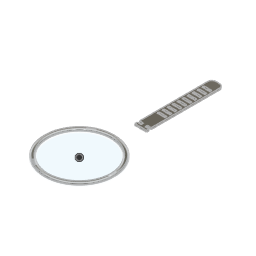
tpuStrapv4 (Autodesk Fusion 360 design; units mm, degrees)
Autodesk Fusion 360 part; units mm, degrees
sketch "Sketch1" plane through (0, 0, 0) normal (0, 0, 1) x (1, 0, 0)
  circle A0 centre (0, 0) radius 40
  circle A1 centre (0, 0) radius 45
  dimension "d1" = 80
  dimension "d3" = 5
  constraint coincident A0.centre A1.centre
  measures "d1" diameter of A0
  measures "d3" distance of A0 A1
extrude "Extrude1" add sketch "Sketch1" along normal blind 3 makes body 1
ref_plane "WorkPlane1" through (60, 0, 0) normal (1, 0, 0) x (0, 1, 0)
sketch "Sketch9" plane through (0, 0, 0) normal (0, 0, 1) x (1, 0, 0)
  circle A0 centre (0, 0) radius 45
  line L0 (-18.1458, 39.7599) -> (-25.3567, 35.5828)
  line L1 (-25.3567, 35.5828) -> (-24.3542, 33.8522)
  line L2 (-24.3542, 33.8522) -> (-17.1433, 38.0293)
  line L3 (-17.1433, 38.0293) -> (-18.1458, 39.7599)
  line L4 (-18.1458, 39.7599) -> (-24.3542, 33.8522) construction
  line L5 (-25.3567, 35.5828) -> (-17.1433, 38.0293) construction
  line L6 (43.5, 4.1667) -> (41.5, 4.1667)
  line L7 (41.5, 4.1667) -> (41.5, -4.1667)
  line L8 (41.5, -4.1667) -> (43.5, -4.1667)
  line L9 (43.5, -4.1667) -> (43.5, 4.1667)
  line L10 (43.5, 4.1667) -> (41.5, -4.1667) construction
  line L11 (41.5, 4.1667) -> (43.5, -4.1667) construction
  line L12 (-17.1416, -38.0234) -> (-18.1416, -39.7554)
  line L13 (-18.1416, -39.7554) -> (-25.3584, -35.5888)
  line L14 (-25.3584, -35.5888) -> (-24.3584, -33.8567)
  line L15 (-24.3584, -33.8567) -> (-17.1416, -38.0234)
  line L16 (-17.1416, -38.0234) -> (-25.3584, -35.5888) construction
  line L17 (-18.1416, -39.7554) -> (-24.3584, -33.8567) construction
  line L18 (0, 0) -> (115, 0)
  line L19 (0, 0) -> (-50, -86.6025)
  line L20 (0, 0) -> (99.9995, 0) construction
  line L21 (0, 0) -> (-50, 86.6025)
  line L22 (0, 0) -> (100, 0) construction
  point P0 (-21.25, 36.8061)
  point P1 (42.5, 0)
  point P2 (-21.25, -36.8061)
  dimension "d44" = 8.3333
  dimension "d45" = 2
  dimension "d46" = 2
  dimension "d47" = 8.3333
  dimension "d48" = 2
  dimension "d49" = 8.3333
  dimension "d108" = 42.5
  dimension "d110" = 42.5
  dimension "d112" = 120
  dimension "d114" = 42.5
  dimension "d115" = 120
  constraint perpendicular L0 L1
  constraint parallel L0 L2
  constraint parallel L1 L3
  constraint coincident L4 P0
  constraint coincident L5 P0
  constraint horizontal L6
  constraint perpendicular L6 L7
  constraint parallel L6 L8
  constraint parallel L7 L9
  constraint coincident L10 P1
  constraint coincident L11 P1
  constraint perpendicular L12 L13
  constraint parallel L12 L14
  constraint parallel L13 L15
  constraint coincident L16 P2
  constraint coincident L17 P2
  constraint coincident A0.centre L18.start
  constraint perpendicular L9 L18
  constraint coincident P1 L18
  constraint horizontal L20
  constraint perpendicular L13 L19
  constraint coincident P2 L19
  constraint horizontal L22
  constraint coincident P0 L21
  measures "d44" distance of L1.end L2.end
  measures "d45" distance of L0.end L1.end
  measures "d46" distance of L7.end L8.end
  measures "d47" distance of L6.end L7.end
  measures "d48" distance of L13.end L14.end
  measures "d49" distance of L12.end L13.end
  measures "d108" distance of P1 A0.centre
  measures "d110" distance of P0 A0.centre
  measures "d112" angle of L19 L20
  measures "d114" distance of P2 A0.centre
  measures "d115" angle of L21 L22
extrude "Extrude3" cut sketch "Sketch9" along normal blind 3 contours L12 L13 L15 L19 | L13 L14 L15 L19 bodies 1
extrude "Extrude4" cut sketch "Sketch9" along normal blind 3 contours L6 L7 L9 L18 | L7 L8 L9 L18 bodies 1
extrude "Extrude5" cut sketch "Sketch9" along normal blind 3 contours L0 L1 L2 L21 | L0 L2 L3 L21 bodies 1
sketch "Sketch10" plane through (0, 0, 0) normal (0, 0, 1) x (1, 0, 0)
  line L0 (15.004, 121.2433) -> (0.004, 121.2433)
  line L1 (0.004, 121.2433) -> (0.004, 124.2433)
  line L2 (0.004, 124.2433) -> (15.004, 124.2433)
  line L3 (15.004, 124.2433) -> (15.004, 121.2433)
  line L4 (10.004, 124.2433) -> (5.004, 124.2433)
  line L5 (5.004, 124.2433) -> (5.004, 127.2433)
  line L6 (5.004, 127.2433) -> (10.004, 127.2433)
  line L7 (10.004, 127.2433) -> (10.004, 124.2433)
  line L8 (15.004, 127.2433) -> (0.004, 127.2433)
  line L9 (0.004, 127.2433) -> (0.004, 214.8433)
  line L10 (5.004, 219.8433) -> (10.004, 219.8433)
  line L11 (15.004, 214.8433) -> (15.004, 127.2433)
  arc A0 (15.004, 214.8433) -> (10.004, 219.8433) centre (10.004, 214.8433) ccw
  arc A1 (5.004, 219.8433) -> (0.004, 214.8433) centre (5.004, 214.8433) ccw
  line L12 (2.504, 147.2433) -> (12.504, 147.2433)
  line L13 (12.504, 147.2433) -> (12.504, 149.6433)
  line L14 (12.504, 149.6433) -> (2.504, 149.6433)
  line L15 (2.504, 149.6433) -> (2.504, 147.2433)
  line L16 (2.504, 147.2433) -> (12.504, 149.6433) construction
  line L17 (12.504, 147.2433) -> (2.504, 149.6433) construction
  line L18 (2.504, 153.6433) -> (12.504, 153.6433)
  line L19 (2.504, 156.0433) -> (2.504, 153.6433)
  line L20 (12.504, 156.0433) -> (2.504, 156.0433)
  line L21 (12.504, 153.6433) -> (12.504, 156.0433)
  line L22 (2.504, 160.0433) -> (12.504, 160.0433)
  line L23 (2.504, 162.4433) -> (2.504, 160.0433)
  line L24 (12.504, 162.4433) -> (2.504, 162.4433)
  line L25 (12.504, 160.0433) -> (12.504, 162.4433)
  line L26 (2.504, 166.4433) -> (12.504, 166.4433)
  line L27 (2.504, 168.8433) -> (2.504, 166.4433)
  line L28 (12.504, 168.8433) -> (2.504, 168.8433)
  line L29 (12.504, 166.4433) -> (12.504, 168.8433)
  line L30 (2.504, 172.8433) -> (12.504, 172.8433)
  line L31 (2.504, 175.2433) -> (2.504, 172.8433)
  line L32 (12.504, 175.2433) -> (2.504, 175.2433)
  line L33 (12.504, 172.8433) -> (12.504, 175.2433)
  line L34 (2.504, 179.2433) -> (12.504, 179.2433)
  line L35 (2.504, 181.6433) -> (2.504, 179.2433)
  line L36 (12.504, 181.6433) -> (2.504, 181.6433)
  line L37 (12.504, 179.2433) -> (12.504, 181.6433)
  line L38 (2.504, 185.6433) -> (12.504, 185.6433)
  line L39 (2.504, 188.0433) -> (2.504, 185.6433)
  line L40 (12.504, 188.0433) -> (2.504, 188.0433)
  line L41 (12.504, 185.6433) -> (12.504, 188.0433)
  line L42 (2.504, 192.0433) -> (12.504, 192.0433)
  line L43 (2.504, 194.4433) -> (2.504, 192.0433)
  line L44 (12.504, 194.4433) -> (2.504, 194.4433)
  line L45 (12.504, 192.0433) -> (12.504, 194.4433)
  line L46 (2.504, 198.4433) -> (12.504, 198.4433)
  line L47 (2.504, 200.8433) -> (2.504, 198.4433)
  line L48 (12.504, 200.8433) -> (2.504, 200.8433)
  line L49 (12.504, 198.4433) -> (12.504, 200.8433)
  line L50 (2.504, 204.8433) -> (12.504, 204.8433)
  line L51 (2.504, 207.2433) -> (2.504, 204.8433)
  line L52 (12.504, 207.2433) -> (2.504, 207.2433)
  line L53 (12.504, 204.8433) -> (12.504, 207.2433)
  point P0 (10.004, 124.2433)
  point P1 (5.004, 124.2433)
  point P2 (10.004, 127.2433)
  point P3 (5.004, 127.2433)
  point P4 (15.004, 219.8433)
  point P5 (7.504, 148.4433)
  point P6 (19.5, 80)
  point P7 (7.504, 148.4433)
  dimension "d56" = 15
  dimension "d57" = 3
  dimension "d58" = 5
  dimension "d59" = 5
  dimension "d61" = 3
  dimension "d77" = 15
  dimension "d78" = 92.6
  dimension "d79" = 5
  dimension "d80" = 5
  dimension "d81" = 10
  dimension "d82" = 2.4
  dimension "d83" = 20
  dimension "d86" = 0
  dimension "d87" = 6.4
  dimension "d88" = 5
  dimension "d89" = 5
  dimension "d92" = 2.5
  constraint horizontal L0
  constraint vertical L1
  constraint horizontal L2
  constraint vertical L3
  constraint coincident L2 P0
  constraint coincident L2 P1
  constraint perpendicular L4 L5
  constraint parallel L4 L6
  constraint parallel L5 L7
  constraint coincident P1 L4.end
  constraint parallel L2 L4
  constraint coincident P0 L4.start
  constraint coincident P2 L6.end
  constraint coincident P3 L5.end
  constraint horizontal L8
  constraint vertical L9
  constraint horizontal L10
  constraint vertical L11
  constraint coincident P4 L10
  constraint coincident P4 L11
  constraint tangent L10 A0
  constraint tangent L11 A0
  constraint tangent L9 A1
  constraint tangent L10 A1
  constraint horizontal L12
  constraint perpendicular L12 L13
  constraint parallel L12 L14
  constraint parallel L13 L15
  constraint coincident L16 P7
  constraint coincident L17 P7
  constraint coincident P7 P5
  measures "d56" distance of L0.start L0.end
  measures "d57" distance of L0.start L2.end
  measures "d58" distance of L3 P0
  measures "d59" distance of L1 P1
  measures "d61" distance of P0 P2
  measures "d77" distance of L8.start L8.end
  measures "d78" distance of L8.start P4
  measures "d79" radius of A0
  measures "d80" radius of A1
  measures "d81" distance of L13.end L14.end
  measures "d82" distance of L12.end L13.end
  measures "d83" distance of L6 L12
  measures "d88" distance of P2 L8.start
  measures "d89" distance of P3 L8.end
  measures "d92" distance of L9 L15
extrude "Extrude6" add sketch "Sketch10" along normal blind 2 separate body contours L6 L8 L9 L10 L11 A0 A1 makes body 2
extrude "Extrude7" add sketch "Sketch10" along normal blind 2 separate body contours L0 L1 L2 L3 L4 | L2 L4 L5 L6 L7 L8 makes body 3
move_face "OffsetFaces3" offset 0.01 3 faces at (6.6707, 127.2433, 0.6667) (3.3373, 127.2433, 0.6667) (13.3373, 127.2433, 0.6667) on bodies 2
combine "Combine5" operation add target body 2 tool bodies 3
fillet "Fillet1" radius 1 1 edges at (-41.9547, -16.2727, 3) on bodies 1
fillet "Fillet2" radius 1 1 edges at (-37.2931, 14.4646, 3) on bodies 1
fillet "Fillet3" radius 1 1 edges at (-41.9547, -16.2727, 0) on bodies 1
fillet "Fillet4" radius 1 1 edges at (-37.2931, 14.4646, 0) on bodies 1
move_body "Move1" bodies 2 to x (1, 0, 0) y (0, 1, 0) z (0, 0, 1) at (0, -50, 0)
equation "d1 = ring_diameter"
equation "d3 = ring_width"
equation "ring_diameter = 80 mm" comment "Diameter of Ring"
equation "ring_width = 5 mm" comment "Width of ring"
equation "strap_start_length = 20 mm" comment "length of strap to first slot"
equation "strap_slot_undersize = 0.6 mm" comment "determines slot size being smaller than notch size of base"
equation "strap_slot_num = 10" comment "Number of slots in straps"
equation "strap_end_length = 15 mm" comment "length of end of strap"
equation "ring_thickness = 3 mm" comment "thickness of ring"
equation "strap_thickness = 2 mm" comment "thickness of strap"
equation "strap_width = 15 mm" comment "width of strap"
equation "notch_size = 3 mm" comment "size of notches of plate"
equation "d24 = ring_thickness"
equation "ring_slot_undersize = 0 mm" comment "slot thickness smaller than strap thickness"
equation "d44 = strap_width / 1.8"
equation "d45 = strap_thickness - ring_slot_undersize"
equation "d46 = strap_thickness - ring_slot_undersize"
equation "d47 = strap_width / 1.8"
equation "d48 = strap_thickness - ring_slot_undersize"
equation "d49 = strap_width / 1.8"
equation "d50 = ring_thickness"
equation "d52 = ring_thickness"
equation "d54 = ring_thickness"
equation "d56 = strap_width"
equation "d58 = strap_width / 3"
equation "d59 = strap_width / 3"
equation "d61 = ring_thickness"
equation "strap_slot_spacing = 4 mm" comment "spacing of slots in the straps"
equation "d77 = strap_width"
equation "d78 = strap_start_length + ( notch_size - strap_slot_undersize + strap_slot_spacing ) * ( strap_slot_num - 1 ) + strap_end_length"
equation "d82 = notch_size - strap_slot_undersize"
equation "d83 = strap_start_length"
equation "d85 = strap_slot_num"
equation "d87 = strap_slot_spacing + notch_size - strap_slot_undersize"
equation "d88 = strap_width / 3"
equation "d89 = strap_width / 3"
equation "d90 = strap_thickness"
equation "d92 = ( strap_width - 10 mm ) / 2"
equation "d93 = strap_thickness"
equation "d108 = ring_diameter / 2 + ring_width / 2"
equation "d110 = d108"
equation "d114 = d108"
